Autodesk Fusion 360 part; units mm, degrees
(part 2 of 2)
  line L285 (-14.2405, -67.8878, 10) -> (-27.2405, -67.8878, 10)
  line L286 (-138.0655, -48.8378, 10) -> (-151.0655, -48.8378, 10)
  arc A286 through (-276.178, -24.7378, 10) (-275.8244, -24.5913, 10) (-275.678, -24.2378, 10)
  line L287 (-142.828, -86.9378, 10) -> (-155.828, -86.9378, 10)
  arc A287 through (-108.703, -124.2503, 10) (-108.5566, -124.6038, 10) (-108.203, -124.7503, 10)
  arc A288 through (-257.128, -24.7378, 10) (-256.7744, -24.5913, 10) (-256.628, -24.2378, 10)
  line L288 (-11.8593, -10.7378, 10) -> (-24.8593, -10.7378, 10)
  line L289 (-103.9405, -43.2878, 10) -> (-103.9405, -30.2878, 10)
  arc A289 through (-22.478, -110.7503, 10) (-22.8316, -110.8967, 10) (-22.978, -111.2503, 10)
  arc A290 through (-76.153, -124.7503, 10) (-75.7994, -124.6038, 10) (-75.653, -124.2503, 10)
  arc A291 through (-22.978, -124.2503, 10) (-22.8316, -124.6038, 10) (-22.478, -124.7503, 10)
  arc A292 through (-270.628, -24.2378, 10) (-270.4816, -24.5913, 10) (-270.128, -24.7378, 10)
  line L290 (-257.715, -99.4378, 10) -> (-257.715, -85.4378, 10)
  line L291 (-142.0405, -43.2878, 10) -> (-142.0405, -30.2878, 10)
  line L292 (-89.653, -81.3878, 10) -> (-89.653, -68.3878, 10)
  line L293 (-232.8155, -62.3378, 10) -> (-232.8155, -49.3378, 10)
  arc A293 through (-161.0905, -43.2878, 10) (-160.9441, -43.6413, 10) (-160.5905, -43.7878, 10)
  line L294 (-156.6155, -62.3378, 10) -> (-156.6155, -49.3378, 10)
  line L295 (-180.928, -100.9378, 10) -> (-193.928, -100.9378, 10)
  arc A294 through (-71.3905, -43.7878, 10) (-71.0369, -43.6413, 10) (-70.8905, -43.2878, 10)
  line L296 (-142.328, -100.4378, 10) -> (-142.328, -87.4378, 10)
  line L297 (-122.9905, -43.2878, 10) -> (-122.9905, -30.2878, 10)
  line L298 (-156.328, -100.4378, 10) -> (-156.328, -87.4378, 10)
  arc A295 through (-263.7718, -49.3378, 10) (-263.9182, -48.9842, 10) (-264.2718, -48.8378, 10)
  line L299 (-137.5655, -124.2503, 10) -> (-137.5655, -111.2503, 10)
  line L300 (-13.7405, -81.3878, 10) -> (-13.7405, -68.3878, 10)
  arc A296 through (-122.4905, -29.7878, 10) (-122.8441, -29.9342, 10) (-122.9905, -30.2878, 10)
  line L301 (-270.628, -124.2503, 10) -> (-270.628, -111.2503, 10)
  line L302 (-295.228, -100.9378, 10) -> (-308.228, -100.9378, 10)
  line L303 (-257.128, -110.7503, 10) -> (-270.128, -110.7503, 10)
  line L304 (-114.253, -110.7503, 10) -> (-127.253, -110.7503, 10)
  line L305 (-238.078, -100.9378, 10) -> (-251.078, -100.9378, 10)
  arc A297 through (-51.053, -67.8878, 10) (-51.4066, -68.0342, 10) (-51.553, -68.3878, 10)
  arc A298 through (-51.553, -81.3878, 10) (-51.4066, -81.7413, 10) (-51.053, -81.8878, 10)
  line L306 (-232.528, -124.2503, 10) -> (-232.528, -111.2503, 10)
  arc A299 through (-286.2098, -61.3378, 10) (-286.0633, -61.6913, 10) (-285.7098, -61.8378, 10)
  arc A300 through (-277.2718, -48.8378, 10) (-277.6253, -48.9842, 10) (-277.7718, -49.3378, 10)
  arc A301 through (-21.3843, -43.7878, 10) (-21.0307, -43.6413, 10) (-20.8843, -43.2878, 10)
  arc A302 through (-255.3338, -47.3378, 10) (-255.4802, -46.9842, 10) (-255.8338, -46.8378, 10)
  line L307 (-195.2155, -124.7503, 10) -> (-208.2155, -124.7503, 10)
  arc A303 through (-108.203, -67.8878, 10) (-108.5566, -68.0342, 10) (-108.703, -68.3878, 10)
  line L308 (-85.678, -86.9378, 10) -> (-98.678, -86.9378, 10)
  arc A304 through (-288.591, -99.4378, 10) (-288.4446, -99.7913, 10) (-288.091, -99.9378, 10)
  arc A305 through (-36.3223, -28.2878, 10) (-36.4687, -27.9342, 10) (-36.8223, -27.7878, 10)
  line L309 (-22.978, -100.4378, 10) -> (-22.978, -87.4378, 10)
  line L310 (-208.7155, -124.2503, 10) -> (-208.7155, -111.2503, 10)
  line L311 (-27.7405, -81.3878, 10) -> (-27.7405, -68.3878, 10)
  arc A306 through (-85.678, -100.9378, 10) (-85.3244, -100.7913, 10) (-85.178, -100.4378, 10)
  arc A307 through (-189.1655, -48.8378, 10) (-189.5191, -48.9842, 10) (-189.6655, -49.3378, 10)
  line L312 (-66.628, -86.9378, 10) -> (-79.628, -86.9378, 10)
  line L313 (-38.053, -67.8878, 10) -> (-51.053, -67.8878, 10)
  arc A308 through (-137.278, -100.4378, 10) (-137.1316, -100.7913, 10) (-136.778, -100.9378, 10)
  line L314 (-175.6655, -124.2503, 10) -> (-175.6655, -111.2503, 10)
  arc A309 through (-99.4655, -49.3378, 10) (-99.6119, -48.9842, 10) (-99.9655, -48.8378, 10)
  arc A310 through (-227.2655, -48.8378, 10) (-227.6191, -48.9842, 10) (-227.7655, -49.3378, 10)
  line L315 (-219.028, -124.7503, 10) -> (-232.028, -124.7503, 10)
  line L316 (-275.678, -124.2503, 10) -> (-275.678, -111.2503, 10)
  arc A311 through (-218.528, -87.4378, 10) (-218.6744, -87.0842, 10) (-219.028, -86.9378, 10)
  line L317 (-47.578, -100.9378, 10) -> (-60.578, -100.9378, 10)
  line L318 (-138.0655, -110.7503, 10) -> (-151.0655, -110.7503, 10)
  arc A312 through (-151.5655, -62.3378, 10) (-151.4191, -62.6913, 10) (-151.0655, -62.8378, 10)
  line L319 (-142.828, -100.9378, 10) -> (-155.828, -100.9378, 10)
  line L320 (-123.778, -100.9378, 10) -> (-136.778, -100.9378, 10)
  arc A313 through (-151.0655, -48.8378, 10) (-151.4191, -48.9842, 10) (-151.5655, -49.3378, 10)
  line L321 (-251.578, -100.4378, 10) -> (-251.578, -87.4378, 10)
  line L322 (-123.778, -86.9378, 10) -> (-136.778, -86.9378, 10)
  arc A314 through (-308.228, -48.8378, 10) (-308.5816, -48.9842, 10) (-308.728, -49.3378, 10)
  arc A315 through (-266.653, -100.9378, 10) (-266.2994, -100.7913, 10) (-266.153, -100.4378, 10)
  line L323 (-157.1155, -124.7503, 10) -> (-170.1155, -124.7503, 10)
  arc A316 through (-189.6655, -62.3378, 10) (-189.5191, -62.6913, 10) (-189.1655, -62.8378, 10)
  arc A317 through (-138.0655, -62.8378, 10) (-137.7119, -62.6913, 10) (-137.5655, -62.3378, 10)
  line L324 (-282.091, -99.9378, 10) -> (-288.091, -99.9378, 10)
  line L325 (-161.878, -86.9378, 10) -> (-174.878, -86.9378, 10)
  arc A318 through (-237.578, -111.2503, 10) (-237.7244, -110.8967, 10) (-238.078, -110.7503, 10)
  line L326 (-47.078, -100.4378, 10) -> (-47.078, -87.4378, 10)
  line L327 (-219.028, -110.7503, 10) -> (-232.028, -110.7503, 10)
  line L328 (-66.128, -100.4378, 10) -> (-66.128, -87.4378, 10)
  line L329 (-281.591, -99.4378, 10) -> (-281.591, -85.4378, 10)
  arc A319 through (-260.603, -67.8878, 10) (-260.9566, -68.0342, 10) (-261.103, -68.3878, 10)
  arc A320 through (-94.4155, -62.3378, 10) (-94.2691, -62.6913, 10) (-93.9155, -62.8378, 10)
  arc A321 through (-218.528, -111.2503, 10) (-218.6744, -110.8967, 10) (-219.028, -110.7503, 10)
  line L330 (-57.103, -67.8878, 10) -> (-70.103, -67.8878, 10)
  arc A322 through (-223.003, -81.3878, 10) (-222.8566, -81.7413, 10) (-222.503, -81.8878, 10)
  line L331 (-276.178, -124.7503, 10) -> (-289.178, -124.7503, 10)
  line L332 (-28.528, -86.9378, 10) -> (-41.528, -86.9378, 10)
  line L333 (-171.403, -81.8878, 10) -> (-184.403, -81.8878, 10)
  line L334 (6, -141.488, 10) -> (6, 6, 10)
  arc A323 through (-61.3655, -49.3378, 10) (-61.5119, -48.9842, 10) (-61.8655, -48.8378, 10)
  arc A324 through (-74.8655, -48.8378, 10) (-75.2191, -48.9842, 10) (-75.3655, -49.3378, 10)
  arc A325 through (-75.653, -68.3878, 10) (-75.7994, -68.0342, 10) (-76.153, -67.8878, 10)
  arc A326 through (-37.553, -68.3878, 10) (-37.6994, -68.0342, 10) (-38.053, -67.8878, 10)
  line L335 (-218.528, -124.2503, 10) -> (-218.528, -111.2503, 10)
  arc A327 through (-189.953, -68.3878, 10) (-190.0994, -68.0342, 10) (-190.453, -67.8878, 10)
  line L336 (-104.728, -86.9378, 10) -> (-117.728, -86.9378, 10)
  arc A328 through (-280.153, -100.4378, 10) (-280.0066, -100.7913, 10) (-279.653, -100.9378, 10)
  arc A329 through (-142.328, -87.4378, 10) (-142.4744, -87.0842, 10) (-142.828, -86.9378, 10)
  line L337 (-114.253, -67.8878, 10) -> (-127.253, -67.8878, 10)
  line L338 (-152.353, -67.8878, 10) -> (-165.353, -67.8878, 10)
  line L339 (-209.503, -67.8878, 10) -> (-222.503, -67.8878, 10)
  line L340 (-209.003, -81.3878, 10) -> (-209.003, -68.3878, 10)
  line L341 (-251.578, -124.2503, 10) -> (-251.578, -111.2503, 10)
  arc A330 through (-203.953, -81.3878, 10) (-203.8066, -81.7413, 10) (-203.453, -81.8878, 10)
  arc A331 through (-288.091, -84.9378, 10) (-288.4446, -85.0842, 10) (-288.591, -85.4378, 10)
  line L342 (-219.028, -24.7378, 10) -> (-232.028, -24.7378, 10)
  line L343 (-80.128, -100.4378, 10) -> (-80.128, -87.4378, 10)
  arc A332 through (-308.228, -86.9378, 10) (-308.5816, -87.0842, 10) (-308.728, -87.4378, 10)
  line L344 (-237.578, -100.4378, 10) -> (-237.578, -87.4378, 10)
  arc A333 through (-232.028, -86.9378, 10) (-232.3816, -87.0842, 10) (-232.528, -87.4378, 10)
  arc A334 through (-194.428, -100.4378, 10) (-194.2816, -100.7913, 10) (-193.928, -100.9378, 10)
  line L345 (-232.528, -100.4378, 10) -> (-232.528, -87.4378, 10)
  line L346 (-189.6655, -124.2503, 10) -> (-189.6655, -111.2503, 10)
  line L347 (-151.5655, -124.2503, 10) -> (-151.5655, -111.2503, 10)
  arc A335 through (-84.4218, -23.7378, 10) (-84.0682, -23.5913, 10) (-83.9218, -23.2378, 10)
  arc A336 through (-108.9905, -30.2878, 10) (-109.1369, -29.9342, 10) (-109.4905, -29.7878, 10)
  line L348 (-257.128, -124.7503, 10) -> (-270.128, -124.7503, 10)
  arc A337 through (-11.8593, -24.7378, 10) (-11.5057, -24.5913, 10) (-11.3593, -24.2378, 10)
  arc A338 through (-43.3223, -42.2878, 10) (-43.1758, -42.6413, 10) (-42.8223, -42.7878, 10)
  line L349 (-114.253, -124.7503, 10) -> (-127.253, -124.7503, 10)
  line L350 (-9.478, -86.9378, 10) -> (-22.478, -86.9378, 10)
  line L351 (-28.028, -100.4378, 10) -> (-28.028, -87.4378, 10)
  arc A339 through (-34.3843, -29.7878, 10) (-34.7378, -29.9342, 10) (-34.8843, -30.2878, 10)
  arc A340 through (-308.728, -43.2878, 10) (-308.5816, -43.6413, 10) (-308.228, -43.7878, 10)
  line L352 (-8.978, -124.2503, 10) -> (-8.978, -111.2503, 10)
  line L353 (-47.578, -86.9378, 10) -> (-60.578, -86.9378, 10)
  arc A341 through (-20.8843, -30.2878, 10) (-21.0307, -29.9342, 10) (-21.3843, -29.7878, 10)
  line L354 (-56.603, -124.2503, 10) -> (-56.603, -111.2503, 10)
  arc A342 through (-227.7655, -62.3378, 10) (-227.6191, -62.6913, 10) (-227.2655, -62.8378, 10)
  arc A343 through (-36.8223, -42.7878, 10) (-36.4687, -42.6413, 10) (-36.3223, -42.2878, 10)
  arc A344 through (-263.4843, -43.2878, 10) (-263.3378, -43.6413, 10) (-262.9843, -43.7878, 10)
  arc A345 through (-223.2905, -30.2878, 10) (-223.4369, -29.9342, 10) (-223.7905, -29.7878, 10)
  arc A346 through (-195.2155, -62.8378, 10) (-194.8619, -62.6913, 10) (-194.7155, -62.3378, 10)
  arc A347 through (-218.2405, -43.2878, 10) (-218.0941, -43.6413, 10) (-217.7405, -43.7878, 10)
  arc A348 through (-55.8155, -48.8378, 10) (-56.1691, -48.9842, 10) (-56.3155, -49.3378, 10)
  line L355 (-138.0655, -124.7503, 10) -> (-151.0655, -124.7503, 10)
  arc A349 through (-122.9905, -43.2878, 10) (-122.8441, -43.6413, 10) (-122.4905, -43.7878, 10)
  line L356 (-195.2155, -110.7503, 10) -> (-208.2155, -110.7503, 10)
  line L357 (-176.1655, -124.7503, 10) -> (-189.1655, -124.7503, 10)
  arc A350 through (-294.728, -49.3378, 10) (-294.8744, -48.9842, 10) (-295.228, -48.8378, 10)
  line L358 (-276.178, -110.7503, 10) -> (-289.178, -110.7503, 10)
  line L359 (-76.153, -110.7503, 10) -> (-89.153, -110.7503, 10)
  line L360 (-57.103, -124.7503, 10) -> (-70.103, -124.7503, 10)
  line L361 (-94.703, -124.2503, 10) -> (-94.703, -111.2503, 10)
  arc A351 through (-151.853, -68.3878, 10) (-151.9994, -68.0342, 10) (-152.353, -67.8878, 10)
  arc A352 through (-204.7405, -43.7878, 10) (-204.3869, -43.6413, 10) (-204.2405, -43.2878, 10)
  line L362 (-123.278, -100.4378, 10) -> (-123.278, -87.4378, 10)
  arc A353 through (-308.228, -29.7878, 10) (-308.5816, -29.9342, 10) (-308.728, -30.2878, 10)
  arc A354 through (-142.0405, -43.2878, 10) (-141.8941, -43.6413, 10) (-141.5405, -43.7878, 10)
  line L363 (-157.1155, -110.7503, 10) -> (-170.1155, -110.7503, 10)
  arc A355 through (-113.753, -68.3878, 10) (-113.8994, -68.0342, 10) (-114.253, -67.8878, 10)
  arc A356 through (-147.5905, -43.7878, 10) (-147.2369, -43.6413, 10) (-147.0905, -43.2878, 10)
  arc A357 through (-294.728, -68.3878, 10) (-294.8744, -68.0342, 10) (-295.228, -67.8878, 10)
  arc A358 through (-232.528, -24.2378, 10) (-232.3816, -24.5913, 10) (-232.028, -24.7378, 10)
  line L364 (-70.603, -124.2503, 10) -> (-70.603, -111.2503, 10)
  line L365 (-194.7155, -124.2503, 10) -> (-194.7155, -111.2503, 10)
  arc A359 through (-128.5405, -43.7878, 10) (-128.1869, -43.6413, 10) (-128.0405, -43.2878, 10)
  dimension "d35" = 329.706
  dimension "d36" = 147.488
  dimension "d37" = 6
  dimension "d38" = 3.5
  dimension "d39" = 3.5
sketch "Sketch4" plane through (0, 0, 13) normal (0, 0, 1) x (-1, 0, 0)
  line L0 (0, -135.488) -> (-317.706, -135.488)
  line L1 (-317.706, -135.488) -> (-317.706, -128.2503)
  line L2 (-317.706, -128.2503) -> (0, -128.2503)
  line L3 (0, -128.2503) -> (0, -135.488)
  line L4 (-9.478, -124.7503) -> (-22.478, -124.7503)
  line L5 (0, -108.2503) -> (-317.706, -108.2503)
  line L6 (-317.706, -108.2503) -> (-317.706, -103.4378)
  line L7 (-317.706, -103.4378) -> (0, -103.4378)
  line L8 (0, -103.4378) -> (0, -108.2503)
  line L9 (0, 0) -> (0, -135.488)
  line L10 (-317.706, -135.488) -> (-317.706, 0)
  line L11 (-9.478, -110.7503) -> (-22.478, -110.7503)
  line L12 (-9.478, -100.9378) -> (-22.478, -100.9378)
  line L13 (0, -135.488) -> (-5.478, -135.488)
  line L14 (-5.478, -135.488) -> (-5.478, 0)
  line L15 (-5.478, 0) -> (0, 0)
  line L16 (0, 0) -> (0, -135.488)
  line L17 (-317.706, 0) -> (0, 0)
  line L18 (-8.978, -124.2503) -> (-8.978, -111.2503)
  line L19 (-317.706, -135.488) -> (-313.728, -135.488)
  line L20 (-313.728, -135.488) -> (-313.728, 0)
  line L21 (-313.728, 0) -> (-317.706, 0)
  line L22 (-317.706, 0) -> (-317.706, -135.488)
  line L23 (-308.728, -24.2378) -> (-308.728, -11.2378)
  line L24 (0, 0) -> (-317.706, 0)
  line L25 (-317.706, 0) -> (-317.706, -5.7378)
  line L26 (-317.706, -5.7378) -> (0, -5.7378)
  line L27 (0, -5.7378) -> (0, 0)
  line L28 (-11.8593, -10.7378) -> (-24.8593, -10.7378)
  line L29 (0, -85.4378) -> (-317.706, -85.4378)
  line L30 (-317.706, -85.4378) -> (-317.706, -80.3878)
  line L31 (-317.706, -80.3878) -> (0, -80.3878)
  line L32 (0, -80.3878) -> (0, -85.4378)
  line L33 (-14.2405, -81.8878) -> (-27.2405, -81.8878)
  line L34 (-9.478, -86.9378) -> (-22.478, -86.9378)
  line L35 (0, -66.3878) -> (-317.706, -66.3878)
  line L36 (-317.706, -66.3878) -> (-317.706, -61.8378)
  line L37 (-317.706, -61.8378) -> (0, -61.8378)
  line L38 (0, -61.8378) -> (0, -66.3878)
  line L39 (-14.2405, -67.8878) -> (-27.2405, -67.8878)
  line L40 (-16.6218, -62.8378) -> (-29.6218, -62.8378)
  line L41 (0, -46.8378) -> (-317.706, -46.8378)
  line L42 (-317.706, -46.8378) -> (-317.706, -42.7878)
  line L43 (-317.706, -42.7878) -> (0, -42.7878)
  line L44 (0, -42.7878) -> (0, -46.8378)
  line L45 (-16.6218, -48.8378) -> (-29.6218, -48.8378)
  line L46 (-21.3843, -43.7878) -> (-34.3843, -43.7878)
  line L47 (0, -27.7878) -> (-317.706, -27.7878)
  line L48 (-317.706, -27.7878) -> (-317.706, -23.7378)
  line L49 (-317.706, -23.7378) -> (0, -23.7378)
  line L50 (0, -23.7378) -> (0, -27.7878)
  line L51 (-12.9463, -27.7878) -> (-18.9463, -27.7878)
  line L52 (-11.8593, -24.7378) -> (-24.8593, -24.7378)
  line L53 (-21.3843, -29.7878) -> (-34.3843, -29.7878)
  line L54 (-24.5, -135.488) -> (-43, -135.488)
  line L55 (-43, -135.488) -> (-43, -128.2503)
  line L56 (-43, -128.2503) -> (-24.5, -128.2503)
  line L57 (-24.5, -128.2503) -> (-24.5, -135.488)
  point P0 (-24.5, -135.488)
  point P1 (-43, -135.488)
  point P2 (-317.706, -135.488)
  point P3 (0, -135.488)
  dimension "d40" = 3.5
  dimension "d41" = 2.5
  dimension "d42" = 2.5
  dimension "d43" = 3.5
  dimension "d44" = 5
  dimension "d45" = 5
  dimension "d46" = 1.5
  dimension "d47" = 1.5
  dimension "d48" = 1.5
  dimension "d49" = 1
  dimension "d50" = 2
  dimension "d51" = 1
  dimension "d53" = 1
  dimension "d54" = 2
  constraint horizontal L0
  constraint vertical L1
  constraint horizontal L2
  constraint vertical L3
  constraint horizontal L5
  constraint vertical L6
  constraint horizontal L7
  constraint vertical L8
  constraint coincident L5.start L9
  constraint coincident L6.end L10
  constraint horizontal L13
  constraint vertical L14
  constraint horizontal L15
  constraint vertical L16
  constraint coincident P3 L0.start
  constraint coincident L14.end L17
  constraint horizontal L19
  constraint vertical L20
  constraint horizontal L21
  constraint vertical L22
  constraint coincident L17 L20.end
  constraint coincident P2 L0.end
  constraint horizontal L24
  constraint vertical L25
  constraint horizontal L26
  constraint vertical L27
  constraint coincident L22 L25.end
  constraint coincident L9.start L15.end
  constraint horizontal L29
  constraint vertical L30
  constraint horizontal L31
  constraint vertical L32
  constraint coincident L22 L30.end
  constraint coincident L9 L29.start
  constraint horizontal L35
  constraint vertical L36
  constraint horizontal L37
  constraint vertical L38
  constraint coincident L22 L36.end
  constraint coincident L16 L35.start
  constraint horizontal L41
  constraint vertical L42
  constraint horizontal L43
  constraint vertical L44
  constraint coincident L10 L42.end
  constraint coincident L16 L41.start
  constraint horizontal L47
  constraint vertical L48
  constraint horizontal L49
  constraint vertical L50
  constraint coincident L22 L48.end
  constraint coincident L9 L47.start
  constraint horizontal L54
  constraint vertical L55
  constraint horizontal L56
  constraint vertical L57
  constraint coincident L2 L55.end
  constraint coincident L0 P0
  measures "d40" distance of L2 L4
  measures "d41" distance of L5 L11
  measures "d42" distance of L7 L12
  measures "d43" distance of L14 L18
  measures "d44" distance of L20 L23
  measures "d45" distance of L26 L28
  measures "d46" distance of L31 L33
  measures "d47" distance of L29 L34
  measures "d48" distance of L35 L39
  measures "d49" distance of L37 L40
  measures "d50" distance of L41 L45
  measures "d51" distance of L43 L46
  measures "d53" distance of L49 L52
  measures "d54" distance of L47 L53
extrude "Extrude5" add sketch "Sketch4" along normal blind 10 from surface at -12.5 contours L0 L2 L3 L9 L13 L14 L16 | L0 L2 L14 L57 | L2 L5 L9 L14 L16 | L5 L7 L8 L9 L14 L16 | L0 L2 L20 L55 | L5 L7 L14 L20 | L7 L9 L14 L16 L29 | L0 L1 L2 L10 L19 L20 L22 | L2 L5 L10 L20 L22 | L5 L6 L7 L10 L20 L22 | L9 L14 L16 L29 L31 L32 | L7 L10 L20 L22 L29 | L14 L20 L29 L31 | L9 L14 L16 L31 L35 | L10 L20 L22 L29 L30 L31 | L9 L14 L16 L35 L37 L38 | L10 L20 L22 L31 L35 | L14 L20 L35 L37 | L9 L14 L16 L37 L41 | L10 L20 L22 L35 L36 L37 | L9 L14 L16 L41 L43 L44 | L10 L20 L22 L37 L41 | L14 L20 L41 L43 | L9 L14 L16 L43 L47 | L10 L20 L22 L41 L42 L43 | L9 L14 L16 L47 L49 L50 | L10 L20 L22 L43 L47 | L14 L20 L47 L49 L51 | L9 L14 L16 L26 L49 | L10 L20 L22 L47 L48 L49 | L9 L14 L15 L16 L17 L24 L26 L27 | L10 L20 L22 L26 L49 | L14 L17 L20 L24 L26 | L10 L17 L20 L21 L22 L24 L25 L26 bodies 1 in component "MechKeyboard"
component "MechKeyboard" placed x (1, 0, 0) y (0, 1, 0) z (0, 0, 1) at (0, 0, 0)
equation "d9 = 17.5 mm - 3.1 mm"
